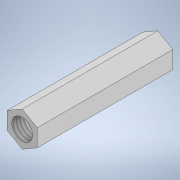
# Autodesk Inventor part: Кусок металла
Saved by Autodesk Inventor 2022 (Build 260153000, 153)
## iProperties
Created: 2022-07-09
Part Number: Кусок металла
Material: Типовые
Document SubType Name: Modeling
Designer: Константин
Density: 1 g/cm^3
Appearance: По умолчанию
Author: Константин
Autodesk Inventor part; units mm, degrees
ref_plane "YZ Plane" through (0, 0, 0) normal (1, 0, 0) x (0, 1, 0)
ref_plane "XZ Plane" through (0, 0, 0) normal (0, 1, 0) x (-1, 0, 0)
ref_plane "XY Plane" through (0, 0, 0) normal (0, 0, 1) x (1, 0, 0)
sketch "Эскиз1" plane through (0, 0, 0) normal (0, 0, 1) x (1, 0, 0)
  line L0 (0, 2.5) -> (2.1651, 1.25)
  line L1 (2.1651, 1.25) -> (2.1651, -1.25)
  line L2 (2.1651, -1.25) -> (0, -2.5)
  line L3 (0, -2.5) -> (-2.1651, -1.25)
  line L4 (-2.1651, -1.25) -> (-2.1651, 1.25)
  line L5 (-2.1651, 1.25) -> (0, 2.5)
  point P0 (0, 0)
  point P1 (0, 0)
  dimension "d0" = 5
  constraints: 12 end point, 1 coincident, 13 other
  measures "d0" distance of L2.end L0.start
extrude "Выдавливание1" add sketch "Эскиз1" against normal blind 19.5
sketch "Эскиз2" plane through (0, 0, 0) normal (0, 0, 1) x (1, 0, 0)
  circle A0 centre (0, 0) radius 1.5
  dimension "d3" = 3
  constraints: 1 centre point, 1 coincident
  measures "d3" diameter of A0
extrude "Выдавливание2" cut sketch "Эскиз2" against normal through all
thread "Резьба1" size "M3x0.5" class "6H" standard "ANSI Metric M Profile" full length
